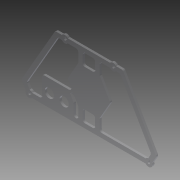
# Autodesk Inventor part: Top Plat
Saved by Autodesk Inventor 2015 (Build 190159000, 159)
## iProperties
Created: 2016-10-14
Part Number: Top Plat
Material: Generic
Document SubType Name: Modeling
Designer: James Yelland
Density: 1 g/cm^3
Appearance: Default
Author: James Yelland
Autodesk Inventor part; units mm, degrees
ref_plane "YZ Plane" through (0, 0, 0) normal (1, 0, 0) x (0, 1, 0)
ref_plane "XZ Plane" through (0, 0, 0) normal (0, 1, 0) x (-1, 0, 0)
ref_plane "XY Plane" through (0, 0, 0) normal (0, 0, 1) x (1, 0, 0)
sketch "Sketch1" plane through (0, 0, 0) normal (0, 1, 0) x (-1, 0, 0)
  circle A0 centre (32.6132, 75.9327) radius 1.6
  circle A1 centre (-32.6132, 75.9327) radius 1.6
  circle A2 centre (80.7596, -11.9856) radius 1.6
  circle A3 centre (-80.7596, -11.9856) radius 1.6
  circle A4 centre (80.7596, -11.9856) radius 5
  circle A5 centre (32.6132, 75.9327) radius 5
  circle A6 centre (-32.6132, 75.9327) radius 5
  circle A7 centre (-80.7596, -11.9856) radius 5
  line L0 (-90.2776, 1.5) -> (-46.4378, 77.4327)
  line L1 (46.4378, 77.4327) -> (90.2776, 1.5)
  line L2 (-83.3494, 1.5) -> (-42.9737, 71.4327)
  line L3 (36.6132, 72.9327) -> (40.3756, 72.9327)
  line L4 (42.9737, 71.4327) -> (83.3494, 1.5)
  line L5 (83.3494, -1.5) -> (80.1615, -7.0215)
  line L6 (85.3577, -10.0215) -> (90.2776, -1.5)
  line L7 (43.8397, 78.9327) -> (36.6132, 78.9327)
  line L8 (-17.4338, 72.9327) -> (-28.6132, 72.9327)
  line L9 (-28.6132, 78.9327) -> (28.6132, 78.9327)
  line L10 (-36.6132, 72.9327) -> (-40.3756, 72.9327)
  line L11 (-36.6132, 78.9327) -> (-43.8397, 78.9327)
  line L12 (-83.3494, -1.5) -> (-80.1615, -7.0215)
  line L13 (-85.3577, -10.0215) -> (-90.2776, -1.5)
  line L14 (-80.7596, -11.9856) -> (-77.7596, -11.9856) construction
  line L15 (76.7596, -14.9856) -> (-76.7596, -14.9856)
  arc A8 (90.2776, -1.5) -> (90.2776, 1.5) centre (87.6795, 0) ccw
  arc A9 (83.3494, -1.5) -> (83.3494, 1.5) centre (80.7513, 0) ccw
  arc A10 (46.4378, 77.4327) -> (43.8397, 78.9327) centre (43.8397, 75.9327) ccw
  arc A11 (42.9737, 71.4327) -> (40.3756, 72.9327) centre (40.3756, 69.9327) ccw
  arc A12 (-43.8397, 78.9327) -> (-46.4378, 77.4327) centre (-43.8397, 75.9327) ccw
  arc A13 (-40.3756, 72.9327) -> (-42.9737, 71.4327) centre (-40.3756, 69.9327) ccw
  arc A14 (-83.3494, 1.5) -> (-83.3494, -1.5) centre (-80.7513, 0) ccw
  arc A15 (-90.2776, 1.5) -> (-90.2776, -1.5) centre (-87.6795, 0) ccw
  line L16 (42.9737, 71.4327) -> (45.4737, 67.1025)
  line L17 (45.4737, 67.1025) -> (48.4737, 61.9064)
  line L18 (-42.9737, 71.4327) -> (-45.4737, 67.1025)
  line L19 (-45.4737, 67.1025) -> (-48.4737, 61.9064)
  line L20 (-23.0235, 72.9327) -> (-26.0235, 72.9327)
  line L21 (-23.0235, 72.9327) -> (-20.0235, 72.9327)
  line L22 (-28.0015, 33.4735) -> (-14.8357, 56.2774)
  line L23 (-5.4338, 56.9735) -> (5.4338, 56.9735)
  line L24 (14.8357, 56.2774) -> (28.0015, 33.4735)
  line L25 (5.4338, 6.9735) -> (-5.4338, 6.9735)
  line L26 (-14.8357, 7.6697) -> (-28.0015, 30.4735)
  line L27 (14.4338, 6.1697) -> (14.4338, -5.9856)
  line L28 (-14.4338, 6.1697) -> (-14.4338, -5.9856)
  line L29 (-8.4338, -5.9856) -> (-8.4338, 3.9735)
  line L30 (8.4338, -5.9856) -> (8.4338, 3.9735)
  line L31 (-14.4338, 57.7774) -> (-14.4338, 69.9327)
  line L32 (-8.4338, 69.9327) -> (-8.4338, 59.9735)
  line L33 (14.4338, 57.7774) -> (14.4338, 69.9327)
  line L34 (8.4338, 69.9327) -> (8.4338, 59.9735)
  arc A16 (14.4338, -5.9856) -> (17.4338, -8.9856) centre (17.4338, -5.9856) ccw
  arc A17 (14.8357, 7.6697) -> (14.4338, 6.1697) centre (17.4338, 6.1697) ccw
  arc A18 (8.4338, 3.9735) -> (5.4338, 6.9735) centre (5.4338, 3.9735) ccw
  arc A19 (-5.4338, 6.9735) -> (-8.4338, 3.9735) centre (-5.4338, 3.9735) ccw
  arc A20 (-14.4338, 6.1697) -> (-14.8357, 7.6697) centre (-17.4338, 6.1697) ccw
  arc A21 (-28.0015, 33.4735) -> (-28.0015, 30.4735) centre (-25.4034, 31.9735) ccw
  arc A22 (28.0015, 30.4735) -> (28.0015, 33.4735) centre (25.4034, 31.9735) ccw
  arc A23 (-14.8357, 56.2774) -> (-14.4338, 57.7774) centre (-17.4338, 57.7774) ccw
  arc A24 (-14.4338, 69.9327) -> (-17.4338, 72.9327) centre (-17.4338, 69.9327) ccw
  arc A25 (5.4338, 56.9735) -> (8.4338, 59.9735) centre (5.4338, 59.9735) ccw
  arc A26 (-8.4338, 59.9735) -> (-5.4338, 56.9735) centre (-5.4338, 59.9735) ccw
  arc A27 (14.4338, 57.7774) -> (14.8357, 56.2774) centre (17.4338, 57.7774) ccw
  line L35 (17.4338, 72.9327) -> (28.6132, 72.9327)
  line L36 (5.4338, 72.9327) -> (-5.4338, 72.9327)
  line L37 (5.4338, -8.9856) -> (-5.4338, -8.9856)
  line L38 (-17.4338, -8.9856) -> (-76.7596, -8.9856)
  arc A28 (5.4338, -8.9856) -> (8.4338, -5.9856) centre (5.4338, -5.9856) ccw
  arc A29 (-8.4338, -5.9856) -> (-5.4338, -8.9856) centre (-5.4338, -5.9856) ccw
  arc A30 (-17.4338, -8.9856) -> (-14.4338, -5.9856) centre (-17.4338, -5.9856) ccw
  arc A31 (-5.4338, 72.9327) -> (-8.4338, 69.9327) centre (-5.4338, 69.9327) ccw
  arc A32 (8.4338, 69.9327) -> (5.4338, 72.9327) centre (5.4338, 69.9327) ccw
  arc A33 (17.4338, 72.9327) -> (14.4338, 69.9327) centre (17.4338, 69.9327) ccw
  circle A34 centre (33.4338, 2.3349) radius 6.25
  circle A35 centre (53.4338, 2.3349) radius 6.25
  line L39 (86.5956, -77.4481) -> (86.5956, -51.4481)
  line L40 (86.5956, -51.4481) -> (74.5956, -51.4481)
  line L41 (-25.4034, 31.9735) -> (-28.8675, 31.9735)
  line L42 (-25.4034, 31.9735) -> (-21.9393, 31.9735) construction
  line L43 (-28.8675, 31.9735) -> (-26.3675, 36.3037)
  line L44 (-26.3675, 36.3037) -> (-54.0335, 52.2766)
  arc A36 (63.4338, 16.6554) -> (60.4338, 19.6554) centre (60.4338, 16.6554) ccw
  line L45 (8.4338, -14.9856) -> (23.4338, -14.9856)
  line L46 (63.4338, 16.6554) -> (63.4338, -5.9856)
  line L47 (21.7557, 16.6554) -> (24.2916, 16.6554)
  line L48 (20.4338, 6.1697) -> (20.4338, -5.9856)
  line L49 (20.8357, 7.6697) -> (25.1576, 15.1554)
  line L50 (28.0015, 30.4735) -> (24.3537, 24.1554)
  line L51 (19.1576, 15.1554) -> (14.8357, 7.6697)
  line L52 (17.4338, -8.9856) -> (17.4338, -8.9856)
  line L53 (66.4338, -8.9856) -> (76.7596, -8.9856)
  arc A37 (17.4338, -8.9856) -> (20.4338, -5.9856) centre (17.4338, -5.9856) ccw
  arc A38 (20.8357, 7.6697) -> (20.4338, 6.1697) centre (23.4338, 6.1697) ccw
  arc A39 (25.1576, 15.1554) -> (24.2916, 16.6554) centre (24.2916, 15.6554) ccw
  arc A40 (21.7557, 16.6554) -> (19.1576, 15.1554) centre (21.7557, 13.6554) ccw
  arc A41 (24.3537, 24.1554) -> (26.9518, 19.6554) centre (26.9518, 22.6554) ccw
  arc A42 (63.4338, -5.9856) -> (66.4338, -8.9856) centre (66.4338, -5.9856) ccw
  line L54 (26.9518, 19.6554) -> (60.4338, 19.6554)
  point P0 (0, 0)
  point P1 (0, 0)
  point P2 (45.5718, 78.9327)
  point P3 (91.1436, 0)
  point P4 (0, 0)
  point P5 (-84.2154, 0)
  point P6 (-42.1077, 72.9327)
  point P7 (-76.7596, -8.9856)
  point P8 (-80.8494, -5.8301)
  point P9 (-74.3148, -8.9856)
  point P10 (80.8494, -5.8301)
  point P11 (74.3148, -8.9856)
  point P12 (-63.1615, 36.4663)
  point P13 (-14.4338, 56.9735)
  point P14 (14.4338, 56.9735)
  point P15 (-14.4338, 6.9735)
  point P16 (-14.4338, -8.9856)
  point P17 (-8.4338, -8.9856)
  point P18 (8.4338, -8.9856)
  point P19 (-8.4338, 72.9327)
  point P20 (14.4338, 72.9327)
  point P21 (8.4338, 72.9327)
  point P22 (20.0236, 16.6554)
  point P23 (26.0236, 16.6554)
  dimension "d0" = 3.2
  dimension "d1" = 3.2
  dimension "d2" = 3.2
  dimension "d3" = 10
  dimension "d4" = 10
  dimension "d24" = 3
  dimension "d27" = 5
  dimension "d29" = 6
  dimension "d31" = 5
  dimension "d33" = 6
  dimension "d36" = 3
  dimension "d37" = 3
  dimension "d39" = 50
  dimension "d44" = 3
  dimension "d45" = 26
  dimension "d46" = 12
  dimension "d47" = 180
  dimension "d48" = 5
  dimension "d49" = 90
  dimension "d54" = 6
  dimension "d56" = 3
  dimension "d57" = 1
  dimension "d58" = 3
  constraints: 108 end point, 83 point on circle, 59 tangent, 43 centre point, 43 point on line, 26 equal radius, 6 coincident, 6 horizontal, 4 collinear, 4 perpendicular, 3 vertical, 2 parallel, 1 midpoint, 15 other
  measures "d0" diameter of A0
  measures "d1" diameter of A2
  measures "d2" diameter of A3
  measures "d3" diameter of A4
  measures "d4" diameter of A5
  measures "d24" radius of A8
  measures "d27" distance of L4.start L16.end
  measures "d29" distance of L16.end L17.end
  measures "d31" distance of L2.end L18.end
  measures "d33" distance of L18.end L19.end
  measures "d36" distance of L20.start L20.end
  measures "d37" distance of L20.start L21.end
  measures "d39" distance between parallel lines of L23 L25
  measures "d44" radius of A28
  measures "d45" distance of L39.start L39.end
  measures "d46" distance of L39.end L40.end
  measures "d47" angle of L41 L42
  measures "d48" distance of L41.end L43.end
  measures "d49" angle of L44 L43
  measures "d54" distance of point (20.024, 16.655) point (26.024, 16.655)
  measures "d56" radius of A37
  measures "d57" radius of A39
  measures "d58" radius of A40
extrude "Extrusion1" add sketch "Sketch1" along normal blind 3 contours A4 | A4 L5 A9 L4 A11 L3 A5 L7 A10 L1 A8 L6 | L15 A7 L38 A30 L28 A20 L26 A21 L22 A23 L31 A24 L8 A6 L9 A5 L35 A33 L33 A27 L24 A22 L50 A41 L54 A36 L46 A42 L53 A4 | A7 | L13 A15 L0 A12 L11 A6 L10 A13 L2 A14 L12 A7 | A5 | A6
body "Solid1"
